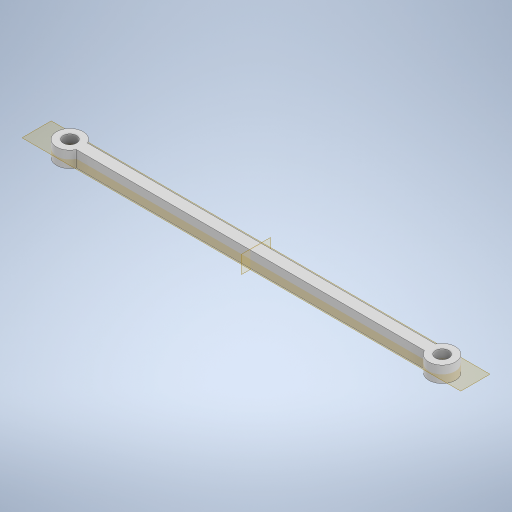
# Autodesk Inventor part: Рычаг
Saved by Autodesk Inventor 2023.2 (Build 272271030, 271C)
## iProperties
Created: 2024-02-06
Part Number: Рычаг
Material: Типовые
Document SubType Name: Modeling
Designer: I9232
Density: 1 g/cm^3
Appearance: По умолчанию
Author: I9232
Autodesk Inventor part; units mm, degrees
ref_plane "XY Plane" through (0, 0, 0) normal (0, 0, 1) x (1, 0, 0)
sketch "Эскиз1" plane through (0, 0, 0) normal (0, 1, 0) x (-1, 0, 0)
  arc A0 (32.7344, -1.057) -> (32.7344, 1.057) centre (35, 0) ccw
  line L0 (32.7344, -1.057) -> (24.3444, -1.057)
  line L1 (30.0057, 0) -> (28.0258, 0)
  line L2 (32.7344, 1.057) -> (24.3444, 1.057)
  circle A1 centre (35, 0) radius 1.25
  line L3 (0, -3.5223) -> (0, 6.6641) construction
  arc A2 (-32.7344, 1.057) -> (-32.7344, -1.057) centre (-35, 0) ccw
  line L4 (-32.7344, -1.057) -> (24.3444, -1.057)
  line L5 (-32.7344, 1.057) -> (24.3444, 1.057)
  circle A3 centre (-35, 0) radius 1.25
  point P0 (0, 0)
  dimension "d2" = 2.5
  dimension "d3" = 35
  dimension "d4" = 2.5
  constraints: 12 end point, 6 symmetric about line, 4 centre point, 4 point on circle, 2 coincident, 2 horizontal, 1 vertical, 2 other
  measures "d2" radius of A0
  measures "d3" distance of point (0, 0) A0.centre
  measures "d4" diameter of A1
extrude "Выдавливание1" add sketch "Эскиз1" along normal mid plane 3
